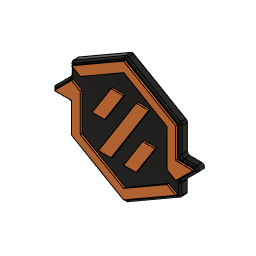
Printed_tophat_Medalion (Autodesk Fusion 360 design; units mm, degrees)
Autodesk Fusion 360 part; units mm, degrees
note: some values were not read from the file. Chosen so that the rebuilt part matches the saved one: which bodies a step acts on. Set by a fixed rule: which sketch regions a step uses.
sketch "Sketch2" plane through (0, 0, 0) normal (0, 1, 0) x (1, 0, 0)
  line L0 (-59.25, -65.792) -> (-59.25, -100)
  line L1 (-59.25, -100) -> (-79, -100)
  line L2 (59.25, -65.792) -> (0, -31.584)
  line L3 (0, -42.9867) -> (49.375, -71.4933)
  line L4 (-49.375, -71.4933) -> (0, -42.9867)
  line L5 (-59.25, -119.75) -> (-49.375, -114.0487)
  line L6 (-79, -100) -> (-59.25, -119.75)
  line L7 (0, -31.584) -> (-59.25, -65.792)
  line L8 (49.375, -71.4933) -> (59.25, -65.792)
  line L9 (-49.375, -114.0487) -> (-49.375, -71.4933)
  line L10 (-49.375, -128.5067) -> (-59.25, -134.208)
  line L11 (59.25, -100) -> (79, -100)
  line L12 (49.375, -128.5067) -> (0, -157.0133)
  line L13 (-59.25, -134.208) -> (0, -168.416)
  line L14 (0, -168.416) -> (59.25, -134.208)
  line L15 (79, -100) -> (59.25, -80.25)
  line L16 (49.375, -85.9513) -> (49.375, -128.5067)
  line L17 (0, -157.0133) -> (-49.375, -128.5067)
  line L18 (59.25, -80.25) -> (49.375, -85.9513)
  line L19 (59.25, -134.208) -> (59.25, -100)
  line L20 (-14.3636, -134.208) -> (-35.9091, -100)
  line L21 (0, -134.208) -> (-14.3636, -134.208)
  line L22 (-35.9091, -100) -> (-21.5455, -100)
  line L23 (-21.5455, -100) -> (0, -134.208)
  line L24 (-28.7273, -65.792) -> (14.3636, -134.208)
  line L25 (-14.3636, -65.792) -> (-28.7273, -65.792)
  line L26 (14.3636, -134.208) -> (28.7273, -134.208)
  line L27 (28.7273, -134.208) -> (-14.3636, -65.792)
  line L28 (35.9091, -100) -> (21.5455, -100)
  line L29 (21.5455, -100) -> (0, -65.792)
  line L30 (0, -65.792) -> (14.3636, -65.792)
  line L31 (14.3636, -65.792) -> (35.9091, -100)
  line L32 (28.7273, -134.208) -> (-28.7273, -65.792) construction
  line L33 (-14.3636, -65.792) -> (14.3636, -134.208) construction
  line L34 (0, -155.5389) -> (0, -174.3649)
  line L35 (0, -172.1688) -> (-62.25, -136.2287)
  line L36 (-62.25, -136.2287) -> (-62.25, -122.2353)
  line L37 (-63.1287, -120.114) -> (-81.1213, -102.1213)
  line L38 (-79, -97) -> (-62.5, -97)
  line L39 (-62.5, -97) -> (-62.5, -63.9156)
  line L40 (0, -25.6351) -> (0, -44.4611)
  line L41 (-62.5, -63.9156) -> (0, -27.8312)
  line L42 (-36, -46.8838) -> (-28, -42.265)
  line L43 (-64, -61.3175) -> (-64, -52.0799)
  line L44 (-28, -157.735) -> (-36, -153.1162)
  arc A0 (-79, -97) -> (-81.1213, -102.1213) centre (-79, -100) ccw
  arc A1 (-62.25, -122.2353) -> (-63.1287, -120.114) centre (-65.25, -122.2353) ccw
  line L45 (0, -27.8312) -> (62.25, -63.7713)
  line L46 (62.25, -63.7713) -> (62.25, -77.7647)
  arc A2 (62.25, -77.7647) -> (63.1287, -79.886) centre (65.25, -77.7647) ccw
  line L47 (63.1287, -79.886) -> (81.1213, -97.8787)
  arc A3 (79, -103) -> (81.1213, -97.8787) centre (79, -100) ccw
  line L48 (79, -103) -> (62.5, -103)
  line L49 (62.5, -103) -> (62.5, -136.0844)
  line L50 (62.5, -136.0844) -> (0, -172.1688)
  point P0 (0, -100)
  dimension "d83" = 1.5
  dimension "d84" = 1.5
  dimension "d85" = 3
  dimension "d86" = 3
  dimension "d87" = 3
  dimension "d88" = 1.5
  dimension "d89" = 3
  dimension "d90" = 3
  dimension "d92" = 360
  constraint midpoint L32 P0
  constraint coincident L34 L35.start
  constraint parallel L13 L35
  constraint vertical L36
  constraint perpendicular L36 L38
  constraint perpendicular L38 L39
  constraint coincident L40 L41.end
  constraint parallel L7 L41
  constraint parallel L6 L37
  constraint tangent L37 A0
  constraint tangent L38 A0
  constraint tangent L36 A1
  constraint tangent L37 A1
  measures "d83" distance of L41 L42
  measures "d84" distance of L39 L43
  measures "d85" distance of L1 L38
  measures "d86" distance of L6 L37
  measures "d87" distance of L5.start L36
  measures "d88" distance of L35 L44
  measures "d89" radius of A0
  measures "d90" radius of A1
extrude "Extrude3" add sketch "Sketch2" against normal blind 8 from surface at 13 contours L0 L1 L4 L5 L6 L7 L9 L40 | L2 L3 L8 L40 | L10 L13 L17 L34 | L11 L12 L14 L15 L16 L18 L19 L34 | L20 L21 L22 L23 | L24 L25 L26 L27 | L28 L29 L30 L31 | L35 L36 L37 L38 L39 L41 A0 A1 L45 L46 A2 L47 A3 L48 L49 L50 makes body 1
extrude "Extrude4" add sketch "Sketch2" against normal blind 2 from surface at 5 contours L0 L1 L4 L5 L6 L7 L9 L40 | L2 L3 L8 L40 | L10 L13 L17 L34 | L11 L12 L14 L15 L16 L18 L19 L34 | L20 L21 L22 L23 | L24 L25 L26 L27 | L28 L29 L30 L31 bodies 1
fillet "Fillet2" radius 3 8 edges at (-62.25, 9, 136.2287) (0, 9, 172.1688) (-62.5, 9, 63.9156) (0, 9, 27.8312) (62.25, 9, 63.7713) (62.5, 9, 103) (62.5, 9, 136.0844) (-62.5, 9, 97) on bodies 1
split "Split1" by plane through (0, 5, 0) normal (0, -1, 0) bodies 1 makes body 2 at (65.8333, 3, 93.4167) makes body 3 at (-65.8333, 3, 106.5833) makes body 4 at (9.5758, 3, 111.4027) makes body 5 at (-23.9394, 3, 111.4027) makes body 6 at (23.9394, 3, 88.5973)
hole "Hole1" at (-6, 13, 157.4591) direction (0, -1, 0) diameter 4.7 depth 7 tip angle 180 bodies 1
hole "Hole2" at (-6, 13, 42.5409) direction (0, -1, 0) diameter 4.7 depth 7 tip angle 180 bodies 1
hole "Hole3" at (-60.6938, 13, 105.5783) direction (0, -1, 0) diameter 4.7 depth 7 tip angle 180 bodies 1
pattern_circular "C-Pattern1" count 2 over 360 about axis through (0, 34.1709, 100) along (0, 1, 0) of "Hole1", "Hole2", "Hole3"
fillet "Fillet3" radius 2 24 edges at (0, 5, 171.7047) (-31.125, 5, 154.1988) (-61.8481, 5, 135.9967) (-62.25, 5, 128.366) (-62.4784, 5, 121.0872) (-72.125, 5, 111.1176) (-81.7716, 5, 98.8519) (-72.25, 5, 97) (-63.3787, 5, 96.1213) (-62.5, 5, 79.8238) (-62.0981, 5, 64.1477) (-31.25, 5, 45.8734) (0, 5, 28.2953) (31.125, 5, 45.8012) (61.8481, 5, 64.0033) (62.25, 5, 71.634) (62.4784, 5, 78.9128) (72.125, 5, 88.8824) (81.7716, 5, 101.1481) (72.25, 5, 103) (63.3787, 5, 103.8787) (62.5, 5, 120.1762) (62.0981, 5, 135.8523) (31.25, 5, 154.1266) on bodies 1
extrude "Extrude1" [suppressed]
extrude "Extrude2" [suppressed]
fillet "Fillet1" [suppressed]
